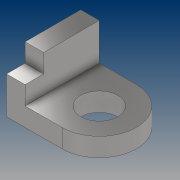
# Autodesk Inventor part: 35
Saved by Autodesk Inventor 2020.2 (Build 242310000, 310)
## iProperties
Created: 2020-09-17
Part Number: 35
Material: 鋼、碳鋼
Document SubType Name: Modeling
Designer: user
Density: 7.85 g/cm^3
Appearance: 半拋光
Mass: 173.812 g
Surface Area: 70.8496 cm^2
Volume: 22.1416 cm^3
Author: user
Autodesk Inventor part; units mm, degrees
ref_plane "YZ Plane" through (0, 0, 0) normal (1, 0, 0) x (0, 1, 0)
ref_plane "XZ Plane" through (0, 0, 0) normal (0, 1, 0) x (-1, 0, 0)
ref_plane "XY Plane" through (0, 0, 0) normal (0, 0, 1) x (1, 0, 0)
sketch "草圖1" plane through (0, 0, 0) normal (0, 1, 0) x (-1, 0, 0)
  circle A0 centre (0, 0) radius 20
  line L0 (0, -20) -> (30, -20)
  line L1 (30, -20) -> (30, 20)
  line L2 (30, 20) -> (0, 20)
  line L3 (0, 20) -> (0, -20)
  point P0 (0, 20)
  dimension "d0" = 40
  dimension "d1" = 30
  constraints: 8 end point, 3 horizontal, 2 parallel, 1 coincident, 1 perpendicular, 3 other
  measures "d1" distance of L0.start L0.end
extrude "擠出1" add sketch "草圖1" along normal blind 30
sketch "草圖2" plane through (-30, 0, 20) normal (0, 0, 1) x (1, 0, 0)
  line L0 (0, 0) -> (0, 30) projected
  line L1 (0, 30) -> (30, 30) projected
  line L2 (30, 0) -> (30, 30) projected
  line L3 (30, 0) -> (0, 0) projected
  line L4 (10, 37.5679) -> (66.1175, 37.5679)
  line L5 (66.1175, 37.5679) -> (66.1175, 10)
  line L6 (66.1175, 10) -> (10, 10)
  line L7 (10, 10) -> (10, 37.5679)
  dimension "d4" = 10
  dimension "d5" = 10
  constraints: 8 end point, 2 parallel, 1 horizontal, 1 perpendicular
  measures "d4" distance between parallel lines of L6 L3
  measures "d5" distance between parallel lines of L7 L0
extrude "擠出2" cut sketch "草圖2" against normal blind 48.25 contours L7 L4 L5 L6 L2 L1 | L1 L2 L6 L7
sketch "草圖3" plane through (-20, 10, 20) normal (1, 0, 0) x (0, 0, -1)
  line L0 (0, 0) -> (40, 0) projected
  line L1 (40, 20) -> (40, 0) projected
  line L2 (0, 20) -> (40, 20) projected
  line L3 (0, 0) -> (0, 20) projected
  line L4 (0, -10) -> (0, 0) projected
  line L5 (40, -10) -> (0, -10) projected
  line L6 (40, 0) -> (40, -10) projected
  line L7 (40, 20) -> (0, 20) projected
  line L8 (0, 20) -> (10, 20)
  line L9 (10, 20) -> (10, 10)
  line L10 (10, 10) -> (0, 10)
  line L11 (0, 10) -> (0, 20)
  point P0 (20, -10)
  dimension "d8" = 10
  dimension "d9" = 10
  constraints: 8 end point, 2 parallel, 1 horizontal, 1 perpendicular
  measures "d8" distance of L9.end L10.end
  measures "d9" distance of L8.end L9.end
extrude "擠出3" cut sketch "草圖3" against normal blind 10 contours L3 L2 L9 L10
sketch "草圖4" plane through (-20, 10, 20) normal (0, 1, 0) x (1, 0, 0)
  arc A0 (20, 0) -> (20, 40) centre (20, 20) ccw projected
  constraints: 1 coincident
hole "孔1" at (0, 10, 0) direction (0, -1, 0) diameter 20 end through all
